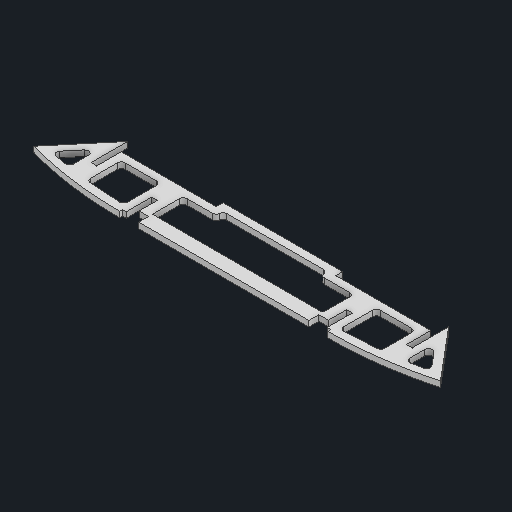
# Autodesk Inventor part: tail_1
Saved by Autodesk Inventor 2023 (Build 270158030, 158C)
## iProperties
Created: 2022-03-21
Part Number: tail_1
Material: Generic
Document SubType Name: Modeling
Designer: kardo
Density: 1 g/cm^3
Appearance: Default
Mass: 8.11511 g
Surface Area: 84.4117 cm^2
Volume: 8.11511 cm^3
Author: kardo
Autodesk Inventor part; units mm, degrees
ref_plane "YZ Plane" through (0, 0, 0) normal (1, 0, 0) x (0, 1, 0)
ref_plane "XZ Plane" through (0, 0, 0) normal (0, 1, 0) x (-1, 0, 0)
ref_plane "XY Plane" through (0, 0, 0) normal (0, 0, 1) x (1, 0, 0)
derived "parameters_frame.ipt"
derived "stencil_frame.ipt"
sketch "sk_joint_locations" plane through (81.12, 0, 0) normal (1, 0, 0) x (0, 1, 0)
  line L0 (0, 0) -> (122.4, 9.6331) construction
  line L1 (36.465, 28.832) -> (112.2, 28.832) construction
  arc A0 (36.465, 28.832) -> (11.22, 28.376) centre (36.465, -670.197) ccw construction
  line L2 (-241.5001, 19.2432) -> (11.22, 28.376) construction
  line L3 (-345, 16.32) -> (-262.2001, 18.586) construction
  arc A1 (-262.2001, 18.586) -> (-241.5001, 19.2432) centre (-326.8578, 2381.2399) ccw construction
  line L4 (-122.4795, 3121.122) -> (270.8781, -1876.9598) construction
  line L5 (-230.0001, 3089.1136) -> (-230.0001, -1866.0023) construction
  line L6 (-114.9999, 3089.1136) -> (-114.9999, -1866.0023) construction
  line L7 (-345, 3089.1136) -> (-345, -1866.0023) construction
  line L8 (0, 3089.1136) -> (0, -1866.0023) construction
  line L9 (529.622, 47.2379) -> (-602.608, 2.7525) construction
  line L10 (-673.1615, -36.5999) -> (647.9226, 67.3717) construction
  line L11 (189.4528, 29.5173) -> (189.1111, 38.2146) construction
  line L12 (201.105, 36.5853) -> (201.7901, 27.8813) construction
  line L13 (0, 14.144) -> (121.9006, 15.9783) construction
  line L14 (-230.0001, 45.8224) -> (-230.0001, 19.6588) construction
  line L15 (-345, 37.3935) -> (-345, 16.32) construction
  line L16 (-114.9999, 50.9907) -> (-114.9999, 23.8147) construction
  line L17 (0, 52.89) -> (0, 27.9705) construction
  line L18 (119.1768, 50.5875) -> (119.7216, 43.6656) construction
  line L19 (120.2663, 36.7438) -> (119.7216, 43.6656) construction
  line L20 (120.2663, 36.7438) -> (120.8111, 29.822) construction
  line L21 (120.8111, 29.822) -> (121.3559, 22.9001) construction
  line L22 (121.3559, 22.9001) -> (121.9006, 15.9783) construction
  line L23 (0, 14.144) -> (0, 0) construction
  spline S0 degree 4 poles (-345, 37.3935) (-258.8686, 45.1235) (-172.5923, 49.7074) (-86.3167, 52.89) (0, 52.89) knots 0 0 0 0 0 1 1 1 1 1
  spline S1 degree 3 poles (0, 52.89) (92.8353, 52.89) (195.0311, 49.5089) (255, 36.448) knots 0 0 0 0 1 1 1 1
  spline S2 degree 2 poles (122.4, 9.6331) (190.08, 14.9596) (255, 36.448) knots 0 0 0 1 1 1
  line L24 (112.2, 37.536) -> (112.2, 28.832) construction
  line L25 (112.2, 35.848) -> (112.2, 30.52) construction
  point P0 (-122.4795, 3121.122)
  point P1 (270.8781, -1876.9598)
  point P2 (189.282, 33.8659)
  point P3 (201.4475, 32.2333)
  point P4 (134.9575, 11.3411)
  point P5 (-345, 26.8568)
  point P6 (-230.0001, 32.7406)
  point P7 (-114.9999, 37.4027)
  point P8 (0, 40.4303)
  point P9 (112.2, 33.184)
sketch "sk_cowl_joint_locations" plane through (54.6, 0, 0) normal (1, 0, 0) x (0, 1, 0)
  line L0 (-345, 16.32) -> (-262.2001, 18.586) construction
  arc A0 (-262.2001, 18.586) -> (-241.5001, 19.2432) centre (-326.8578, 2381.2399) ccw construction
  line L1 (-241.5001, 19.2432) -> (11.22, 28.376) construction
  arc A1 (36.465, 28.832) -> (11.22, 28.376) centre (36.465, -670.197) ccw construction
  line L2 (36.465, 28.832) -> (112.2, 28.832) construction
  line L3 (94.8, 29.632) -> (36.465, 29.632) construction
  arc A2 (36.465, 29.632) -> (11.1911, 29.1755) centre (36.465, -670.197) ccw construction
  line L4 (11.1911, 29.1755) -> (-241.529, 20.0427) construction
  arc A3 (-262.222, 19.3857) -> (-241.529, 20.0427) centre (-326.8578, 2381.2399) ccw construction
  line L5 (-262.222, 19.3857) -> (-345, 17.1203) construction
  line L6 (-230.0001, 3089.1136) -> (-230.0001, -1866.0023) construction
  line L7 (-114.9999, 3089.1136) -> (-114.9999, -1866.0023) construction
  line L8 (-345, 3089.1136) -> (-345, -1866.0023) construction
  line L9 (0, 3089.1136) -> (0, -1866.0023) construction
  line L10 (-230.0001, 44.8681) -> (-230.0001, 20.4593) construction
  line L11 (-114.9999, 49.7658) -> (-114.9999, 24.6152) construction
  line L12 (-345, 17.1203) -> (-345, 17.1203)
  line L13 (-345, 17.1203) -> (-345, 36.7228) construction
  line L14 (-850.7464, 3011.9134) -> (325.2296, -1886.3794) construction
  line L15 (-344.7454, 36.7228) -> (-345, 39.712) construction
  line L16 (0, 51.4) -> (0, 28.7711) construction
  spline S0 degree 2 poles (-345, 39.712) (-172.656, 54.3934) (0, 54.4) knots 0 0 0 1 1 1
  spline S1 degree 3 poles (0, 54.4) (37.026, 54.4) (80.784, 47.9917) (112.2, 37.536) knots 1 1 1 1 2 2 2 2
  spline S2 degree 3 poles (111.2526, 34.6895) (106.0906, 36.4075) (96.4401, 39.2282) (84.5011, 42.0313) (75.2591, 43.9395) (68.9709, 45.1125) (60.9945, 46.449) (54.5373, 47.4124) (46.413, 48.4791) (39.8882, 49.2203) (31.7426, 50.0013) (25.2514, 50.5076) (17.2112, 50.9875) (9.2661, 51.3118) (3.0567, 51.4) (0, 51.4) knots 1 1 1 1 1.166667 1.291667 1.333333 1.416667 1.458333 1.541667 1.583333 1.666667 1.708333 1.791667 1.833333 1.916667 2 2 2 2
  spline S3 degree 3 poles (0, 51.4) (-19.1698, 51.3993) (-52.712, 51.1604) (-91.0357, 50.4121) (-119.7742, 49.6473) (-138.931, 49.0355) (-162.8744, 48.1436) (-182.0269, 47.3282) (-205.9648, 46.1816) (-225.113, 45.1626) (-249.0455, 43.7615) (-268.1894, 42.5387) (-292.1166, 40.883) (-316.041, 39.1) (-335.1777, 37.5379) (-344.7454, 36.7228) knots 0 0 0 0 0.166667 0.291667 0.333333 0.416667 0.458333 0.541666 0.583333 0.666666 0.708333 0.791666 0.833333 0.916666 1 1 1 1
  line L17 (-144.5331, 44.6212) -> (-139.5174, 23.7292) construction
  line L18 (-134.9371, 30.3529) -> (-140.7713, 28.9522) construction
  line L19 (-137.4449, 40.7989) -> (-143.2792, 39.3982) construction
  line L20 (-144.5331, 44.6212) -> (-138.6989, 46.0219) construction
  line L21 (-139.5174, 23.7292) -> (-133.6831, 25.1299) construction
  line L22 (-138.6989, 46.0219) -> (-138.9044, 52.0184) construction
  point P0 (0, 0)
  point P1 (-345, 26.9216)
  point P2 (-230.0001, 32.6637)
  point P3 (-114.9999, 37.1905)
  point P4 (0, 40.0855)
  point P5 (-850.7464, 3011.9134)
  point P6 (325.2296, -1886.3794)
  point P7 (-85.2629, 50.788)
  point P8 (0, 40.0855)
sketch "sk_tail_1_base" plane through (0, -114.9999, 0) normal (0, 1, 0) x (-1, 0, 0)
  spline S0 degree 2 poles (-156, 24.53) (-108.1936, 52.767) (-54.6, 52.767) knots 0 0 0 1 1 1 construction
  line L0 (-54.6, 52.767) -> (0, 52.767) construction
  line L1 (0, -1866.0023) -> (0, 3089.1136) construction
  line L2 (890.9668, -1145.0693) -> (-1640.9022, 1872.2947) construction
  line L3 (-106.5246, 44.9392) -> (-84.12, 18.2385)
  line L4 (-84.12, 18.2385) -> (-84.12, 37.4027)
  line L5 (-84.12, 37.4027) -> (-81.12, 37.4027)
  line L6 (-81.12, 37.4027) -> (-81.12, 24.6147)
  line L7 (-81.12, 24.6147) -> (-31.32, 24.6147)
  line L8 (-31.32, 24.6147) -> (-31.32, 21.0065)
  line L9 (-31.32, 21.0065) -> (0, 21.0065)
  line L10 (0, 21.0065) -> (0, 51.967)
  line L11 (-54.6, 51.967) -> (0, 51.967)
  spline S1 degree 5 poles (-155.5931, 23.8412) (-146.3701, 29.2888) (-136.824, 34.1884) (-126.9698, 38.4699) (-106.9196, 45.5907) (-86.0824, 49.8843) (-75.6273, 51.2855) (-65.1137, 51.9669) (-54.6, 51.967) knots 0 0 0 0 0 0 0.504662 0.504662 0.504662 1 1 1 1 1 1
  point P0 (0, 0)
  point P1 (-34.32, 23.8147)
  point P2 (-34.32, 20.2065)
  dimension "d8" = 0.8
  dimension "d3" = 0.8
  dimension "d4" = 0.8
  dimension "d5" = 3
  dimension "d6" = 3
  dimension "d7" = 0.8
  constraints: 18 end point, 5 parallel, 3 perpendicular, 2 point on line, 4 other
  measures "d3" distance from line of point (-34.32, 20.206) L9
  measures "d4" distance from line of L7 point (-34.32, 23.815)
  measures "d5" distance from line of point (-34.32, 23.815) L8
  measures "d6" distance of L4.end L5.end
  measures "d7" distance between parallel lines of L2 L3
extrude "thicken" add sketch "sk_tail_1_base" along normal blind 3
sketch "sk_cut_stringer_cowl" plane through (0, -114.9999, 0) normal (0, 1, 0) x (-1, 0, 0)
  line L0 (-54.6, -1866.0023) -> (-54.6, 3089.1136) construction
  line L1 (-54.6, 52.767) -> (0, 52.767) projected
  line L2 (-49.6, 52.767) -> (-49.6, 37.1905)
  line L3 (-49.6, 37.1905) -> (-52.6, 37.1905)
  line L4 (-52.6, 37.1905) -> (-52.6, 52.767)
  point P0 (0, 0)
  point P1 (-54.6, 37.1905)
  dimension "d11" = 3
  dimension "d12" = 5
  constraints: 6 end point, 3 point on line, 2 parallel
  measures "d11" distance between parallel lines of L4 L2
  measures "d12" distance between parallel lines of L0 L2
extrude "cut_joint" cut sketch "sk_cut_stringer_cowl" along normal through all both and the other way through all
sketch "sk_cut_cowl_liner" plane through (0, -114.9999, 0) normal (0, 1, 0) x (-1, 0, 0)
  line L0 (-54.6, 52.767) -> (0, 52.767) projected
  line L1 (-54.6, -1866.0023) -> (-54.6, 3089.1136) projected
  line L2 (-44.6, 52.767) -> (-44.6, 46.767)
  line L3 (-44.6, 46.767) -> (-49.6, 46.767)
  line L4 (-49.6, 46.767) -> (-49.6, 50.467)
  line L5 (-49.6, 50.467) -> (-54.6, 50.467)
  point P0 (0, 0)
  dimension "d15" = 5
  dimension "d16" = 5
  dimension "d17" = 2.3
  dimension "d38" = 6
  constraints: 8 end point, 4 parallel, 2 point on line
  measures "d15" distance between parallel lines of L4 L2
  measures "d16" distance of L4.end L5.end
  measures "d17" distance between parallel lines of L0 L5
  measures "d38" distance of L2.start L2.end
extrude "cut_liner" cut sketch "sk_cut_cowl_liner" along normal through all both and the other way through all
sketch "sk_cut_weight" plane through (0, -114.9999, 0) normal (0, 1, 0) x (-1, 0, 0)
  line L0 (-31.32, 21.0065) -> (0, 21.0065) construction
  line L1 (-31.32, 24.6147) -> (-31.32, 21.0065) construction
  line L2 (-81.12, 24.6147) -> (-31.32, 24.6147) construction
  line L3 (-81.12, 37.4027) -> (-81.12, 24.6147) construction
  line L4 (-49.6, 46.767) -> (-49.6, 50.467) construction
  line L5 (-44.6, 46.767) -> (-49.6, 46.767) construction
  line L6 (-44.6, 52.767) -> (-44.6, 46.767) construction
  spline S0 degree 3 poles (-155.5931, 23.8412) (-152.9466, 25.4044) (-147.6273, 28.4002) (-140.9123, 31.8189) (-134.1479, 34.9932) (-128.6969, 37.337) (-121.8335, 40.0224) (-116.3031, 41.9753) (-109.3405, 44.1723) (-103.7306, 45.7345) (-96.6683, 47.4431) (-90.9785, 48.6147) (-82.3837, 50.0792) (-70.8169, 51.5113) (-60.5314, 51.967) (-54.6, 51.967) knots 0 0 0 0 0.083333 0.166667 0.208333 0.291667 0.333333 0.416667 0.458333 0.541667 0.583333 0.666667 0.708333 0.833333 1 1 1 1 construction
  line L7 (0, -1866.0023) -> (0, 3089.1136) projected
  line L8 (0, 25.0065) -> (-27.32, 25.0065)
  line L9 (-27.32, 25.0065) -> (-27.32, 28.6147)
  line L10 (-27.32, 28.6147) -> (-44.6, 28.6147)
  line L11 (-77.12, 28.6147) -> (-77.12, 46.6862)
  line L12 (-77.12, 46.6862) -> (-56.6, 47.967)
  line L13 (-56.6, 47.967) -> (-56.6, 28.6147)
  line L14 (-56.6, 28.6147) -> (-77.12, 28.6147)
  line L15 (-44.6, 44.767) -> (-44.6, 28.6147)
  line L16 (-44.6, 44.767) -> (0, 44.767)
  line L17 (-77.12, 46.6862) -> (-77.12, 50.6862) construction
  line L18 (-49.6, 46.767) -> (-49.6, 24.6147) construction
  line L19 (-49.6, 46.767) -> (-52.6, 46.767) construction
  line L20 (-52.6, 46.767) -> (-52.6, 24.6147) construction
  line L21 (-106.5246, 44.9392) -> (-84.12, 18.2385) construction
  line L22 (-84.12, 18.2385) -> (-84.12, 37.4027) construction
  line L23 (-88.12, 29.2284) -> (-88.12, 45.0962)
  line L24 (-88.12, 45.0962) -> (-99.6847, 43.0107)
  line L25 (-99.6847, 43.0107) -> (-88.12, 29.2284)
  line L26 (-88.12, 45.0962) -> (-88.12, 49.0962) construction
  line L27 (-99.6847, 43.0107) -> (-102.2559, 46.0749) construction
  point P0 (0, 0)
  dimension "d21" = 4
  dimension "d22" = 3
  dimension "d23" = 4
  dimension "d24" = 4
  dimension "d25" = 4
  dimension "d27" = 2
  dimension "d28" = 4
  dimension "d29" = 4
  dimension "d30" = 4
  dimension "d31" = 4
  dimension "d35" = 4
  dimension "d36" = 4
  dimension "d37" = 4
  constraints: 36 end point, 12 parallel, 5 collinear, 4 point on line, 1 equal length, 1 perpendicular, 3 other
  measures "d21" distance of L11.end L17.end
  measures "d22" distance between parallel lines of L20 L18
  measures "d23" distance between parallel lines of L0 L8
  measures "d24" distance between parallel lines of L1 L9
  measures "d25" distance between parallel lines of L10 L2
  measures "d27" distance between parallel lines of L16 L5
  measures "d28" distance between parallel lines of L20 L13
  measures "d29" distance between parallel lines of L2 L14
  measures "d30" distance between parallel lines of L11 L3
  measures "d31" vertical distance of point (-54.6, 51.967) L12.end
  measures "d35" distance between parallel lines of L21 L25
  measures "d36" distance between parallel lines of L23 L22
  measures "d37" distance of L23.end L26.end
extrude "cut_weight" cut sketch "sk_cut_weight" along normal through all both and the other way through all
fillet "round_corners" radius 2 10 edges at (27.32, -113.4999, 25.0065) (27.32, -113.4999, 28.6147) (77.12, -113.4999, 28.6147) (56.6, -113.4999, 28.6147) (44.6, -113.4999, 28.6147) (77.12, -113.4999, 46.6862) (56.6, -113.4999, 47.967) (99.6847, -113.4999, 43.0107) (88.12, -113.4999, 29.2284) (88.12, -113.4999, 45.0962)
mirror "mirror" about plane through (0, 0, 0) normal (1, 0, 0)
equation "\"d8\" = shell_thickness"
equation "\"d3\" = shell_thickness"
equation "\"d4\" = shell_thickness"
equation "\"d5\" = bulkhead_thickness"
equation "\"d6\" = stringer_thickness"
equation "\"d7\" = shell_thickness"
equation "\"d9\" = bulkhead_thickness"
equation "\"d11\" = bulkhead_thickness"
equation "\"d12\" = cowl_liner_width"
equation "\"d15\" = cowl_sealing_width"
equation "\"d16\" = cowl_liner_width"
equation "\"d17\" = shell_thickness + cowl_liner_thickness"
equation "\"d38\" = cowl_sealing_thickness + cowl_shell_thickness + cowl_liner_thickness"
equation "\"d21\" = bulkhead_inset"
equation "\"d22\" = bulkhead_thickness"
equation "\"d23\" = bulkhead_inset"
equation "\"d24\" = bulkhead_inset"
equation "\"d25\" = bulkhead_inset"
equation "\"d28\" = bulkhead_inset"
equation "\"d29\" = bulkhead_inset"
equation "\"d30\" = bulkhead_inset"
equation "\"d31\" = bulkhead_inset"
equation "\"d35\" = bulkhead_inset"
equation "\"d36\" = bulkhead_inset"
equation "\"d37\" = bulkhead_inset"
equation "\"d34\" = 0.5 * bulkhead_inset"
equation "\"shell_thickness\" = 0.8"
equation "\"stringer_thickness\" = 3"
equation "\"bulkhead_thickness\" = 3"
equation "\"cowl_liner_width\" = 5"
equation "\"cowl_sealing_width\" = 5"
equation "\"cowl_liner_thickness\" = 1.5"
equation "\"cowl_sealing_thickness\" = 3"
equation "\"cowl_shell_thickness\" = 1.5"
equation "\"bulkhead_inset\" = 4"
body "Solid1"
